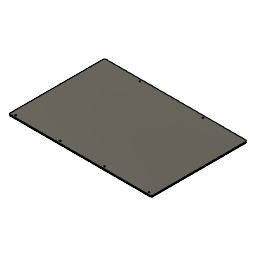
ThirdPlate (Autodesk Fusion 360 design; units mm, degrees)
part number: 2026-09-01-01-07-29-658
part number: 2026-09-01-01-07-30-153
Autodesk Fusion 360 part; units mm, degrees
sketch "Cut_Profile_1to1_QTY1" plane through (0, 0, 0) normal (0, 0, 1) x (1, 0, 0) in component "ThirdPlate"
  line L0 (-178.5, -122) -> (178.5, -122)
  arc A0 (178.5, -122) -> (181.5, -119) centre (178.5, -119) ccw
  line L1 (181.5, -119) -> (181.5, 119)
  arc A1 (181.5, 119) -> (178.5, 122) centre (178.5, 119) ccw
  line L2 (178.5, 122) -> (-178.5, 122)
  arc A2 (-178.5, 122) -> (-181.5, 119) centre (-178.5, 119) ccw
  line L3 (-181.5, 119) -> (-181.5, -119)
  arc A3 (-181.5, -119) -> (-178.5, -122) centre (-178.5, -119) ccw
  circle A4 centre (-86.5, 116) radius 1.6
  circle A5 centre (74.5, 116) radius 1.6
  circle A6 centre (-169.5, -116) radius 1.6
  circle A7 centre (-56.5, -116) radius 1.6
  circle A8 centre (56.5, -116) radius 1.6
  circle A9 centre (169.5, -116) radius 1.6
extrude "Acrylic_Plate_3mm" add sketch "Cut_Profile_1to1_QTY1" along normal blind 3 in component "ThirdPlate"
component "ThirdPlate" placed x (1, 0, 0) y (0, 1, 0) z (0, 0, 1) at (0, 0, 0)
equation "plateLength = 363.0 mm" comment "Finished plate length"
equation "plateWidth = 244.0 mm" comment "Finished plate width"
equation "acrylicThickness = 3.0 mm" comment "Acrylic sheet thickness"
equation "cornerRadius = 3.0 mm" comment "Outside corner radius"
equation "mountHoleDiameter = 3.2 mm" comment "M3 screw clearance-hole diameter"
equation "newTopHoleOffsetTop = 6 mm" comment "New M3 hole centers from top edge"
equation "newTopHole1OffsetLeft = 95 mm" comment "New left M3 hole center from left edge"
equation "newTopHole2OffsetRight = 107 mm" comment "New right M3 hole center from right edge"
equation "bottomMountOffsetLeft = 12 mm" comment "Leftmost bottom M3 center from left edge"
equation "bottomMountOffsetRight = 12 mm" comment "Rightmost bottom M3 center from right edge"
equation "bottomMountOffsetBottom = 6 mm" comment "Bottom M3 centers from bottom edge"
equation "bottomMountSpacing = 113 mm" comment "Spacing between bottom M3 centers"
equation "d13 = acrylicThickness"
named bodies: "ThirdPlate_QTY1"
